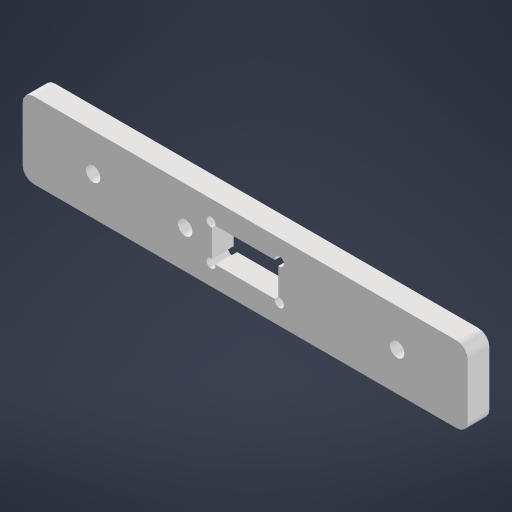
# Autodesk Inventor part: zig9
Saved by Autodesk Inventor 2024.3 (Build 283343000, 343)
## iProperties
Created: 2024-09-11
Part Number: zig9
Material: 일반
Document SubType Name: Modeling
Designer: ASUS
Density: 1 g/cm^3
Appearance: 기본값
Author: ASUS
Autodesk Inventor part; units mm, degrees
ref_plane "YZ Plane" through (0, 0, 0) normal (1, 0, 0) x (0, 1, 0)
ref_plane "XZ Plane" through (0, 0, 0) normal (0, 1, 0) x (-1, 0, 0)
ref_plane "XY Plane" through (0, 0, 0) normal (0, 0, 1) x (1, 0, 0)
ref_plane "작업 평면1" through (0, 0, 0) normal (0, 0, 1) x (1, 0, 0)
sketch "스케치1" plane through (0, 0, 0) normal (0, 0, 1) x (1, 0, 0)
  line L0 (-12, 0) -> (0, 0) projected
  line L1 (0, 0) -> (0, 6) projected
  line L2 (-12, 6) -> (0, 6) projected
  line L3 (-12, 0) -> (-12, 6) projected
  line L4 (0.3, -0.3) -> (-12.3, -0.3)
  line L5 (-12.3, -0.3) -> (-12.3, 6.3)
  line L6 (-12.3, 6.3) -> (0.3, 6.3)
  line L7 (0.3, 6.3) -> (0.3, -0.3)
  line L8 (4, -4) -> (-16, -4)
  line L9 (-16, -4) -> (-16, 10)
  line L10 (-16, 10) -> (4, 10)
  line L11 (4, 10) -> (4, -4)
  line L12 (1, 6) -> (1, 0) projected
  line L13 (1, 0) -> (31, 0) projected
  line L14 (31, 0) -> (31, 6) projected
  line L15 (1, 6) -> (31, 6) projected
  circle A0 centre (22, 3.1) radius 1.35 projected
  line L16 (-13, 0) -> (-13, 6) projected
  line L17 (-43, 6) -> (-13, 6) projected
  line L18 (-43, 0) -> (-43, 6) projected
  line L19 (-43, 0) -> (-13, 0) projected
  circle A1 centre (-34, 3.1) radius 1.35 projected
  line L20 (31, 0) -> (-43, 0)
  line L21 (-43, 0) -> (-43, 6)
  line L22 (-43, 6) -> (31, 6)
  line L23 (31, 6) -> (31, 0)
  line L24 (-47, -4) -> (35, -4)
  line L25 (35, -4) -> (35, 10)
  line L26 (35, 10) -> (-47, 10)
  line L27 (-47, 10) -> (-47, -4)
  circle A2 centre (0.3, 6.3) radius 1.05
  circle A3 centre (0.3, -0.3) radius 1.05
  circle A4 centre (-12.3, -0.3) radius 1.05
  circle A5 centre (-12.3, 6.3) radius 1.05
  point P0 (0.3, 5.25)
  point P1 (0.3, 0.75)
  point P2 (-0.75, -0.3)
  point P3 (-11.25, -0.3)
  point P4 (-12.3, 0.75)
  point P5 (-12.3, 5.25)
  point P6 (-11.25, 6.3)
  point P7 (-0.75, 6.3)
  dimension "d0" = 0.3
  dimension "d1" = 4
  dimension "d4" = 2.1
  dimension "d5" = 2.1
  dimension "d6" = 2.1
  dimension "d7" = 2.1
  constraints: 32 end point, 4 centre point, 4 parallel, 2 perpendicular, 1 coincident, 1 horizontal, 9 other
  measures "d0" distance between parallel lines of L0 L4
  measures "d1" distance between parallel lines of L0 L8
  measures "d4" diameter of A2
  measures "d5" diameter of A3
  measures "d6" diameter of A4
  measures "d7" diameter of A5
extrude "돌출1" add sketch "스케치1" along normal blind 4 contours L4 A3 L13 L11 L8 L9 L19 A4 | A4 L16 A5 L5 | L19 L9 L17 A5 L16 A4 | L7 A2 L12 A3 | L19 L18 L17 L9 | L9 L24 L27 L26 L17 L18 L19 | A5 L17 L9 L10 L11 L15 A2 L6 | L12 A2 L15 L11 L13 A3 | L13 L14 L15 L11 L26 L25 L24 | L11 L15 L14 L13
sketch "스케치2" plane through (0, 0, 4) normal (0, 0, 1) x (1, 0, 0)
  line L0 (-13, 6) -> (-13, 0) projected
  line L1 (-42, 0) -> (-13, 0) projected
  line L2 (-42, 6) -> (-42, 0) projected
  line L3 (-42, 6) -> (-13, 6) projected
  circle A0 centre (-17.05, 3) radius 1.35 projected
  point P0 (0, 0)
extrude "돌출2" cut sketch "스케치2" against normal through all contours A0
fillet "모깎기1" radius 2 4 edges at (35, 10, 2) (35, -4, 2) (-47, 10, 2) (-47, -4, 2)
sketch "스케치3" plane through (0, 0, 4) normal (0, 0, 1) x (1, 0, 0)
  circle A0 centre (-17.05, 3) radius 1.35 projected
  arc A1 (-47, -2) -> (-45, -4) centre (-45, -2) ccw projected
  line L0 (-45, -4) -> (33, -4) projected
  arc A2 (33, -4) -> (35, -2) centre (33, -2) ccw projected
  line L1 (35, -2) -> (35, 8) projected
  arc A3 (35, 8) -> (33, 10) centre (33, 8) ccw projected
  line L2 (33, 10) -> (-45, 10) projected
  arc A4 (-45, 10) -> (-47, 8) centre (-45, 8) ccw projected
  line L3 (-47, 8) -> (-47, -2) projected
  circle A5 centre (22, 3.1) radius 1.35 projected
  circle A6 centre (-34, 3.1) radius 1.35 projected
  arc A7 (0.3, 5.25) -> (-0.75, 6.3) centre (0.3, 6.3) ccw projected
  line L4 (0.3, 5.25) -> (0.3, 0.75) projected
  arc A8 (-0.75, -0.3) -> (0.3, 0.75) centre (0.3, -0.3) ccw projected
  line L5 (-0.75, -0.3) -> (-11.25, -0.3) projected
  arc A9 (-12.3, 0.75) -> (-11.25, -0.3) centre (-12.3, -0.3) ccw projected
  line L6 (-12.3, 0.75) -> (-12.3, 5.25) projected
  arc A10 (-11.25, 6.3) -> (-12.3, 5.25) centre (-12.3, 6.3) ccw projected
  line L7 (-11.25, 6.3) -> (-0.75, 6.3) projected
  line L8 (0.1, 0.5261) -> (0.1, 5.4739)
  arc A11 (0.1, 5.4739) -> (-0.5261, 6.1) centre (0.3, 6.3) ccw
  line L9 (-0.5261, 6.1) -> (-11.4739, 6.1)
  arc A12 (-11.4739, 6.1) -> (-12.1, 5.4739) centre (-12.3, 6.3) ccw
  line L10 (-12.1, 5.4739) -> (-12.1, 0.5261)
  arc A13 (-12.1, 0.5261) -> (-11.4739, -0.1) centre (-12.3, -0.3) ccw
  line L11 (-11.4739, -0.1) -> (-0.5261, -0.1)
  arc A14 (-0.5261, -0.1) -> (0.1, 0.5261) centre (0.3, -0.3) ccw
  point P0 (0, 0)
  dimension "d11" = 0.2
  constraints: 8 end point, 8 point on circle, 4 centre point, 7 other
  measures "d11" distance between parallel lines of L4 L8
extrude "돌출3" add sketch "스케치3" against normal up to surface (4 mm away) contours L4 A8 L5 A9 L6 A10 L7 A7
